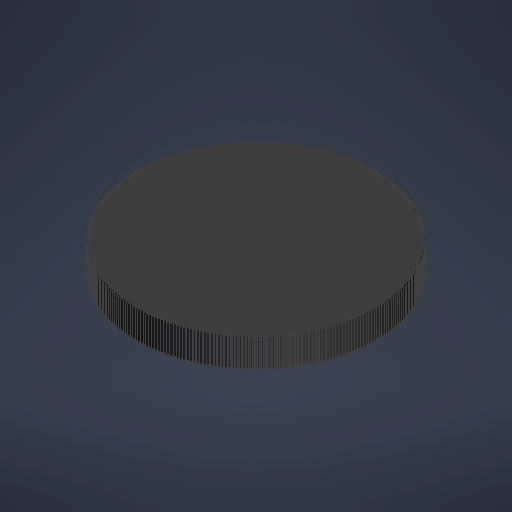
# Autodesk Inventor part: FrostyCarbonCoin25t-Edge
Saved by Autodesk Inventor 2026.1 (Build 301233020, 233B)
## iProperties
Created: 2026-01-02
Part Number: FrostyCarbonCoin25t-Edge
Material: Generic
Document SubType Name: Modeling
Designer: incep
Density: 1 g/cm^3
Appearance: Default
Author: incep
## iProperties of the stored document FrostyCarbonCoin25t-Edge_3DPrint.ipt
Created: 2026-01-03
Part Number: FrostyCarbonCoin25t-Edge_3DPrint
Material: Generic
Document SubType Name: Modeling
Designer: incep
Density: 1 g/cm^3
Appearance: Default
Author: incep
Autodesk Inventor part; units mm, degrees
ref_plane "YZ Plane" through (0, 0, 0) normal (1, 0, 0) x (0, 1, 0)
ref_plane "XZ Plane" through (0, 0, 0) normal (0, 1, 0) x (-1, 0, 0)
ref_plane "XY Plane" through (0, 0, 0) normal (0, 0, 1) x (1, 0, 0)
sketch "Sketch1" plane through (0, 0, 0) normal (0, 1, 0) x (-1, 0, 0)
  circle A0 centre (0, 0) radius 19
  dimension "d0" = 38
  constraints: 1 centre point, 1 coincident
  measures "d0" diameter of A0
sketch "Sketch2" plane through (0, 0, 0) normal (0, 1, 0) x (-1, 0, 0)
  point P0 (0, 0)
extrude "Extrusion1" add sketch "Sketch1" along normal blind 4.5
sketch "Sketch3" plane through (0, 4.5, 0) normal (0, 1, 0) x (1, 0, 0)
  circle A0 centre (0, 0) radius 19 projected
  circle A1 centre (0, 0) radius 18
  dimension "d3" = 1
  constraints: 1 centre point
  measures "d3" radial gap between concentric circles of A0 A1
extrude "Extrusion2" [suppressed]
sketch "Sketch4" plane through (0, 4.5, 0) normal (0, 1, 0) x (1, 0, 0)
  circle A0 centre (0, 0) radius 19 projected
  line L0 (-0.2309, 19) -> (0.2309, 19)
  line L1 (-0.2309, 19) -> (0, 18.6)
  line L2 (0, 18.6) -> (0.2309, 19)
  point P0 (0, 19)
  point P1 (0.2301, 18.9986)
  point P2 (-0.2301, 18.9986)
  dimension "d6" = 60
  dimension "d7" = 0.4
  constraints: 6 end point, 2 vertical alignment, 1 horizontal, 1 midpoint, 1 tangent
  measures "d6" angle of L2 L1
  measures "d7" distance of L1.end point (0, 19)
extrude "Extrusion3" cut sketch "Sketch4" against normal up to surface (4.5 mm away) contours L2 L1 A0 picked at (0, 18.8666)
pattern_circular "Circular Pattern1" count 288 over 360 about axis through (0, -10, 0) along (0, 1, 0) of "Extrusion3"
body "Solid1"
